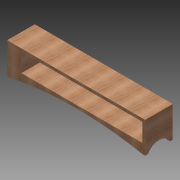
# Autodesk Inventor part: initial sketch
Saved by Autodesk Inventor 2015 (Build 190159000, 159)
## iProperties
Created: 2017-01-31
Part Number: initial sketch
Material: Wood (Birch)
Document SubType Name: Modeling
Designer: jwillauer
Density: 0.55 g/cm^3
Appearance: Birch - Natural Polished
Author: jwillauer
Autodesk Inventor part; units mm, degrees
ref_plane "YZ Plane" through (0, 0, 0) normal (1, 0, 0) x (0, 1, 0)
ref_plane "XZ Plane" through (0, 0, 0) normal (0, 1, 0) x (-1, 0, 0)
ref_plane "XY Plane" through (0, 0, 0) normal (0, 0, 1) x (1, 0, 0)
sketch "Sketch1" plane through (0, 0, 0) normal (0, 0, 1) x (1, 0, 0)
  line L0 (-705.7948, 239.9372) -> (1326.2052, 239.9372)
  line L1 (1326.2052, 239.9372) -> (1326.2052, -217.2628)
  line L2 (1326.2052, -217.2628) -> (-705.7948, -217.2628)
  line L3 (-705.7948, -217.2628) -> (-705.7948, 239.9372)
  point P0 (0, 0)
  dimension "d0" = 2032
  dimension "d1" = 457.2
  constraints: 8 end point, 2 parallel, 1 horizontal, 1 perpendicular
  measures "d0" distance of L0.start L0.end
  measures "d1" distance of L2.end L0.start
extrude "Extrusion1" add sketch "Sketch1" along normal blind 406.4
sketch "Sketch2" plane through (0, 0, 406.4) normal (0, 0, 1) x (1, 0, 0)
  line L0 (-705.7948, -217.2628) -> (1326.2052, -217.2628) projected
  arc A0 (1288.1052, -217.2628) -> (-667.6948, -217.2628) centre (310.2052, -5068.164) ccw
  point P0 (0, 0)
  dimension "d4" = 38.1
  dimension "d5" = 38.1
  constraints: 2 point on circle, 2 point on line, 1 centre point
  measures "d4" distance of L0.start A0.end
  measures "d5" distance of L0.end A0.start
extrude "Extrusion2" cut sketch "Sketch2" against normal blind 406.4
sketch "Sketch4" plane through (1326.2052, -217.2628, 0) normal (1, 0, 0) x (0, 0, -1)
  line L0 (-406.4, 457.2) -> (-406.4, 0) projected
  line L1 (-406.4, 79.0993) -> (0, 97.5865)
  line L2 (-406.4, 97.5865) -> (0, 97.5865) projected
  line L3 (-406.4, 0) -> (-368.3, 0)
  line L4 (0, 0) -> (-406.4, 0) projected
  line L5 (0, 0) -> (-38.1, 0)
  arc A0 (-38.1, 0) -> (-368.3, 0) centre (-203.2, -90.8674) ccw
  point P0 (0, 217.2628)
  dimension "d11" = 38.1
  dimension "d12" = 38.1
  constraints: 6 end point, 4 point on line, 2 point on circle, 1 centre point, 1 tangent
  measures "d11" distance of L0.end L3.end
  measures "d12" distance of L4.start L5.end
extrude "Extrusion3" cut sketch "Sketch4" against normal through all contours A0 L1 | L1 A0 L4
sketch "Sketch5" plane through (0, 0, 406.4) normal (0, 0, 1) x (1, 0, 0)
  line L0 (1281.7552, 195.4872) -> (-496.2448, 195.4872)
  line L1 (-496.2448, 195.4872) -> (-496.2448, -75.2262)
  line L2 (-496.2448, -75.2262) -> (1281.7552, -75.2262)
  line L3 (1281.7552, -75.2262) -> (1281.7552, 195.4872)
  line L4 (-705.7948, 239.9372) -> (-705.7948, -217.2628) projected
  line L5 (1326.2052, 239.9372) -> (-705.7948, 239.9372) projected
  arc A0 (1288.1052, -217.2628) -> (-667.6948, -217.2628) centre (310.2052, -5068.164) ccw projected
  line L6 (310.2052, -119.6762) -> (1461.347, -119.6762)
  line L7 (1326.2052, -217.2628) -> (1326.2052, 239.9372) projected
  point P0 (0, 0)
  dimension "d16" = 44.45
  dimension "d18" = 44.45
  dimension "d19" = 1778
  dimension "d21" = 44.45
  constraints: 10 end point, 2 horizontal, 2 parallel, 1 perpendicular, 1 point on circle, 1 tangent
  measures "d16" distance between parallel lines of L5 L0
  measures "d18" distance between parallel lines of L2 L6
  measures "d19" distance of L0.start L0.end
  measures "d21" distance between parallel lines of L7 L3
extrude "Extrusion4" cut sketch "Sketch5" against normal blind 361.95
sketch "Sketch6" plane through (-705.7948, -217.2628, 0) normal (-1, 0, 0) x (0, 0, 1)
  line L0 (406.4, 142.0365) -> (44.45, 142.0365) projected
  line L1 (44.45, 412.75) -> (361.95, 412.75)
  line L2 (361.95, 412.75) -> (361.95, 142.0365)
  line L3 (361.95, 142.0365) -> (44.45, 142.0365)
  line L4 (44.45, 142.0365) -> (44.45, 412.75)
  line L5 (406.4, 457.2) -> (406.4, 0) projected
  point P0 (0, 217.2628)
  dimension "d24" = 44.45
  constraints: 8 end point, 2 parallel, 1 horizontal, 1 perpendicular, 1 point on line
  measures "d24" distance between parallel lines of L5 L2
extrude "Extrusion5" cut sketch "Sketch6" against normal blind 203.2
body "Solid1"
